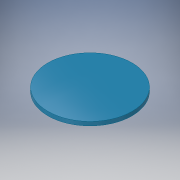
# Autodesk Inventor part: stamp_circular_hand
Saved by Autodesk Inventor 2019 (Build 230136000, 136)
## iProperties
Created: 2019-02-20
Part Number: stamp_circular_hand
Material: PET Plastic
Document SubType Name: Modeling
Designer: jmc
Density: 1.541 g/cm^3
Appearance: Sky Blue Dark
Author: jmc
## iProperties of the stored document stamp_circular_hand_3DPrint.ipt
Created: 2019-02-20
Part Number: stamp_circular_hand_3DPrint
Material: Generic
Document SubType Name: Modeling
Designer: jmc
Density: 1 g/cm^3
Appearance: Default
Author: jmc
Autodesk Inventor part; units mm, degrees
ref_plane "YZ Plane" through (0, 0, 0) normal (1, 0, 0) x (0, 1, 0)
ref_plane "XZ Plane" through (0, 0, 0) normal (0, 1, 0) x (-1, 0, 0)
sketch "Sketch1" plane through (0, 0, 0) normal (0, 1, 0) x (-1, 0, 0)
  circle A0 centre (0, 0) radius 14.91
  dimension "d0" = 29.82
  constraints: 1 centre point, 1 coincident
  measures "d0" diameter of A0
extrude "Extrusion1" add sketch "Sketch1" against normal blind 1.4
ref_plane "Work Plane1" through (0, -1.4, 0) normal (0, 1, 0) x (-1, 0, 0)
sketch "Sketch2" plane through (0, -1.4, 0) normal (0, 1, 0) x (-1, 0, 0)
  line L0 (7.6891, 7.5378) -> (7.6891, -7.5378) construction
  line L1 (7.6891, -7.5378) -> (-7.6891, -7.5378) construction
  line L2 (-7.6891, -7.5378) -> (-7.6891, 7.5378) construction
  line L3 (-7.6891, 7.5378) -> (7.6891, 7.5378) construction
  circle A0 centre (0, 0) radius 14.91 construction
  line L4 (0, 14.91) -> (0, -14.91) construction
  line L5 (-14.91, 0) -> (14.91, 0) construction
  circle A1 centre (0, 0) radius 12.393
  circle A2 centre (0, 0) radius 11.993
  spline S0 degree 2 poles (0, -7.0107) (-2.9061, -7.0107) (-7.0107, -2.9061) (-7.0107, 0) knots 0 0 0 1 2 2 2
  spline S1 degree 2 poles (-7.0107, 0) (-7.0107, 2.9061) (-2.9061, 7.0107) (0, 7.0107) knots 0 0 0 1 2 2 2
  spline S2 degree 2 poles (0, 7.0107) (2.9061, 7.0107) (7.0107, 2.9061) (7.0107, 0) knots 0 0 0 1 2 2 2
  spline S3 degree 2 poles (7.0107, 0) (7.0107, -2.9061) (2.9061, -7.0107) (0, -7.0107) knots 0 0 0 1 2 2 2
  line L6 (4.4341, 3.4454) -> (-3.4454, -4.4341)
  spline S4 degree 2 poles (-3.4454, -4.4341) (-1.8475, -5.6125) (0.01, -5.6125) knots 0 0 0 1 1 1
  spline S5 degree 2 poles (0.01, -5.6125) (2.3369, -5.6125) (5.6125, -2.3369) (5.6125, -0.01) knots 0 0 0 1 2 2 2
  spline S6 degree 2 poles (5.6125, -0.01) (5.6125, 1.8376) (4.4341, 3.4454) knots 0 0 0 1 1 1
  line L7 (-4.4341, -3.4454) -> (3.4454, 4.4341)
  spline S7 degree 2 poles (3.4454, 4.4341) (1.8375, 5.6125) (0, 5.6125) knots 0 0 0 1 1 1
  spline S8 degree 2 poles (0, 5.6125) (-2.3269, 5.6125) (-5.6125, 2.3269) (-5.6125, 0.01) knots 0 0 0 1 2 2 2
  spline S9 degree 2 poles (-5.6125, 0.01) (-5.6125, -1.8875) (-4.4341, -3.4454) knots 0 0 0 1 1 1
  dimension "d5" = 29.82
  dimension "d6" = 15.0756
  dimension "d7" = 15.3782
  dimension "d8" = 7.3722
  dimension "d9" = 7.2209
  dimension "d10" = 0.4
  constraints: 4 end point, 4 point on circle, 2 centre point, 1 perpendicular, 1 vertical, 2 other
  measures "d5" diameter of A0
  measures "d6" distance of L1.end L2.end
  measures "d7" distance of L0.end L1.end
  measures "d8" distance from line of L4.start L3
  measures "d9" distance from line of L5.start L2
  measures "d10" radial gap between concentric circles of A1 A2
extrude "Extrusion2" add sketch "Sketch2" against normal blind 0.4
equation "\"d8\" = 0.5 * d5 - 0.5 * d6"
equation "\"d9\" = 0.5 * d5 - 0.5 * d7"
body "Solid1"
